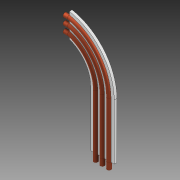
# Autodesk Inventor part: 1123B_Top Heat Sink Mirror_V1
Saved by Autodesk Inventor 2020 (Build 240168000, 168)
## iProperties
Created: 2019-10-13
Part Number: 1123B_Top Heat Sink Mirror_V1
Material: Aluminum
Document SubType Name: Modeling
Designer: RFLab
Density: 2.7 g/cm^3
Appearance: Satin
Author: RFLab
Autodesk Inventor part; units mm, degrees
ref_plane "YZ Plane" through (0, 0, 0) normal (1, 0, 0) x (0, 1, 0)
ref_plane "XZ Plane" through (0, 0, 0) normal (0, 1, 0) x (-1, 0, 0)
ref_plane "XY Plane" through (0, 0, 0) normal (0, 0, 1) x (1, 0, 0)
sketch "Sketch1" plane through (0, 0, 0) normal (0, 0, 1) x (1, 0, 0)
  circle A0 centre (0, 0) radius 75 construction
  circle A1 centre (0, 0) radius 130 construction
  line L0 (-130, 0) -> (-130, -130)
  line L1 (-75, 0) -> (-75, -130)
  line L2 (-75, -130) -> (-130, -130)
  line L3 (0, 0) -> (-25, 0) construction
  line L4 (-25, 0) -> (-25, 130) construction
  line L5 (-25, 130) -> (0, 130) construction
  line L6 (0, 130) -> (0, 0) construction
  arc A2 (-25, 127.5735) -> (-130, 0) centre (0, 0) ccw
  arc A3 (-25, 70.7107) -> (-75, 0) centre (0, 0) ccw
  line L7 (-25, 70.7107) -> (-25, 127.5735)
  dimension "d0" = 150
  dimension "d1" = 55
  dimension "d2" = 130
  dimension "d3" = 25
  constraints: 16 end point, 9 point on circle, 4 centre point, 3 vertical, 2 concentric, 2 parallel, 2 perpendicular, 2 point on line, 2 tangent, 1 coincident, 1 horizontal
  measures "d0" diameter of A0
  measures "d1" radial gap between concentric circles of A0 A1
  measures "d2" distance of L0.start L0.end
  measures "d3" distance of L4.end L5.end
extrude "Extrusion1" add sketch "Sketch1" along normal blind 6.35
sketch "Sketch2" plane through (-25, 70.7107, 0) normal (1, 0, 0) x (0, 0, -1)
  line L0 (-6.35, 0) -> (-6.35, 56.8628) projected
  circle A0 centre (-6.35, 12) radius 4.7625
  circle A1 centre (-6.35, 28.4314) radius 4.7625
  circle A2 centre (-6.35, 44.8628) radius 4.7625
  point P0 (0, -70.7107)
  dimension "d6" = 9.525
  dimension "d7" = 9.525
  dimension "d8" = 9.525
  dimension "d9" = 12
  dimension "d10" = 12
  constraints: 3 centre point, 2 point on line, 1 midpoint
  measures "d6" diameter of A0
  measures "d7" diameter of A1
  measures "d8" diameter of A2
  measures "d9" distance of L0.start A0.centre
  measures "d10" distance of L0.end A2.centre
sketch "Sketch5" plane through (0, 0, 6.35) normal (0, 0, 1) x (1, 0, 0)
  line L0 (-130, 0) -> (-130, -130) projected
  line L1 (-75, -130) -> (-75, 0) projected
  line L2 (-130, 0) -> (-75, 0)
  line L3 (-130, -130) -> (-75, -130) projected
  line L4 (-118, -130) -> (-118, 0)
  line L5 (-102.5, -130) -> (-102.5, 0)
  line L6 (-87, -130) -> (-87, 0)
  arc A0 (-25, 115.5735) -> (-118, 0) centre (0.3131, 0) ccw
  arc A1 (-25, 99.1421) -> (-102.5, 0) centre (-0.3361, 0) ccw
  arc A2 (-25, 82.7107) -> (-87, 0) centre (-0.8302, 0) ccw
  line L7 (-118, -130) -> (-118, -143.1393)
  line L8 (-102.5, -130) -> (-102.5, -141.8458)
  line L9 (-87, -130) -> (-87, -139.9056)
  point P0 (0, 0)
  dimension "d16" = 12
  dimension "d17" = 12
  constraints: 14 end point, 6 point on circle, 4 point on line, 3 centre point, 3 tangent, 3 vertical, 2 midpoint, 2 perpendicular, 1 horizontal
  measures "d16" distance of L0.end L4.start
  measures "d17" distance from line of L1 L6.start
sweep "Sweep2" cut profiles "Sketch2" path "Sketch5" path curves A2 L6 L9 contours A0 L0 | L0 A0
sweep "Sweep3" cut profiles "Sketch2" path "Sketch5" path curves A1 L5 L8 contours A1 L0 | L0 A1
sweep "Sweep4" cut profiles "Sketch2" path "Sketch5" path curves A0 L4 L7 contours A2 L0 | L0 A2
sketch "Sketch6" plane through (-25, 70.7107, 0) normal (1, 0, 0) x (0, 0, -1)
  arc A0 (-6.35, 7.2375) -> (-6.35, 16.7625) centre (-6.35, 12) ccw construction
  arc A1 (-6.35, 23.6689) -> (-6.35, 33.1939) centre (-6.35, 28.4314) ccw construction
  arc A2 (-6.35, 40.1003) -> (-6.35, 49.6253) centre (-6.35, 44.8628) ccw construction
  circle A3 centre (-6.35, 12) radius 4.7625
  circle A4 centre (-6.35, 28.4314) radius 4.7625
  line L0 (-6.35, 33.1939) -> (-6.35, 40.1003) projected
  circle A5 centre (-6.35, 44.8628) radius 4.7625
  circle A6 centre (-6.35, 12) radius 4.2625
  circle A7 centre (-6.35, 28.4314) radius 4.2625
  circle A8 centre (-6.35, 44.8628) radius 4.2625
  point P0 (0, -70.7107)
  dimension "d24" = 0.5
  dimension "d25" = 0.5
  dimension "d26" = 0.5
  constraints: 3 centre point, 3 coincident, 3 vertical alignment, 6 other
sweep "Sweep5" add profiles "Sketch6" path "Sketch5" separate body path curves A2 L6 L9 contours A3
sweep "Sweep6" add profiles "Sketch6" path "Sketch5" separate body path curves A1 L5 L8 contours A4
sweep "Sweep7" add profiles "Sketch6" path "Sketch5" separate body path curves A0 L4 L7 contours A5
sketch "Sketch7" plane through (-130, -130, 0) normal (0, -1, 0) x (1, 0, 0)
  line L0 (55, 0) -> (0, 0)
  line L1 (0, 0) -> (0, 25)
  line L2 (0, 25) -> (55, 25)
  line L3 (55, 25) -> (55, 0)
  point P0 (130, 0)
  dimension "d33" = 25
  dimension "d34" = 55
  constraints: 8 end point, 2 parallel, 1 horizontal, 1 perpendicular
  measures "d33" distance of L0.end L1.end
  measures "d34" distance of L1.end L2.end
extrude "Extrusion2" cut sketch "Sketch7" along normal through all bodies 2 3 4
sketch "Sketch8" plane through (-130, -130, 0) normal (0, -1, 0) x (1, 0, 0)
  ellipse E0 centre (12, 6.35) end of major axis (12, 10.6125) minor radius 4.1638 projected
  ellipse E1 centre (12, 6.35) end of major axis (12, 1.5875) minor radius 4.6522 projected
  point P0 (130, 0)
  constraints: 2 other
extrude "Extrusion3" add sketch "Sketch8" along normal blind 15 bodies 2
sketch "Sketch9" plane through (-130, -130, 0) normal (0, -1, 0) x (1, 0, 0)
  ellipse E0 centre (27.5, 6.35) end of major axis (27.5, 10.6125) minor radius 4.1364 projected
  ellipse E1 centre (27.5, 6.35) end of major axis (27.5, 1.5875) minor radius 4.6216 projected
  point P0 (130, 0)
  constraints: 2 other
extrude "Extrusion4" add sketch "Sketch9" along normal blind 15 bodies 2
sketch "Sketch10" plane through (-130, -130, 0) normal (0, -1, 0) x (1, 0, 0)
  ellipse E0 centre (43, 6.35) end of major axis (43, 10.6125) minor radius 4.0914 projected
  ellipse E1 centre (43, 6.35) end of major axis (43, 1.5875) minor radius 4.5713 projected
  point P0 (130, 0)
  constraints: 2 other
extrude "Extrusion5" add sketch "Sketch10" along normal blind 15 bodies 2
sketch "Sketch11" plane through (-25, 82.7107, 6.35) normal (1, 0, 0) x (0, 0, -1)
  circle A0 centre (0, 0) radius 4.2625 projected
  circle A1 centre (0, 0) radius 4.7625 projected
  point P0 (6.35, -82.7107)
  point P1 (4.2625, 0)
  point P2 (4.7625, 0)
  constraints: 2 horizontal alignment
extrude "Extrusion6" add sketch "Sketch11" along normal blind 10 bodies 2
sketch "Sketch12" plane through (-25, 99.1421, 6.35) normal (1, 0, 0) x (0, 0, -1)
  circle A0 centre (0, 0) radius 4.2625 projected
  circle A1 centre (0, 0) radius 4.7625 projected
  point P0 (6.35, -99.1421)
  point P1 (4.2625, 0)
  point P2 (4.7625, 0)
  constraints: 2 horizontal alignment
extrude "Extrusion7" add sketch "Sketch12" along normal blind 10 bodies 3
sketch "Sketch13" plane through (-25, 115.5735, 6.35) normal (1, 0, 0) x (0, 0, -1)
  circle A0 centre (0, 0) radius 4.2625 projected
  circle A1 centre (0, 0) radius 4.7625 projected
  point P0 (6.35, -115.5735)
  point P1 (4.2625, 0)
  point P2 (4.7625, 0)
  constraints: 2 horizontal alignment
extrude "Extrusion8" add sketch "Sketch13" along normal blind 10 bodies 4
mirror "Mirror1" about plane through (-25, 70.7107, 0) normal (1, 0, 0) remove original yes bodies 4 1 3 2
equation "\"d10\" = d9"
equation "\"d16\" = d9"
equation "\"d17\" = d16"
body "Solid1"
body "Solid2"
body "Solid3"
body "Solid4"
